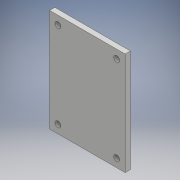
# Autodesk Inventor part: placa trasera
Saved by Autodesk Inventor 2017 (Build 210142000, 142)
## iProperties
Part Number: placa trasera
Material: Genérico
Document SubType Name: Modeling
Designer: user
Density: 1 g/cm^3
Appearance: Valor por defecto
Author: user
Autodesk Inventor part; units mm, degrees
ref_plane "YZ Plane" through (0, 0, 0) normal (1, 0, 0) x (0, 1, 0)
ref_plane "XZ Plane" through (0, 0, 0) normal (0, 1, 0) x (-1, 0, 0)
ref_plane "XY Plane" through (0, 0, 0) normal (0, 0, 1) x (1, 0, 0)
sketch "Boceto1" plane through (0, 0, 0) normal (0, 1, 0) x (-1, 0, 0)
  line L0 (36, -49) -> (-36, -49)
  line L1 (-36, -49) -> (-36, 49)
  line L2 (-36, 49) -> (36, 49)
  line L3 (36, 49) -> (36, -49)
  point P0 (0, 0)
  point P1 (0, -49)
  point P2 (-36, 0)
  dimension "d0" = 72
  dimension "d1" = 98
  constraints: 8 end point, 2 midpoint, 2 parallel, 1 horizontal, 1 horizontal alignment, 1 perpendicular, 1 vertical alignment
  measures "d0" distance of L1.end L2.end
  measures "d1" distance of L2.end L0.start
extrude "Extrusión1" add sketch "Boceto1" along normal blind 5
sketch "Boceto2" plane through (0, 5, 0) normal (0, 1, 0) x (1, 0, 0)
  point P0 (-28, -41)
  point P1 (28, -41)
  point P2 (28, 41)
  point P3 (-28, 41)
hole "Agujero1" at (-28, 5, 41) at (28, 5, 41) at (28, 5, -41) at (-28, 5, -41) direction (0, -1, 0) diameter 5.5 depth 5
